Autodesk Fusion 360 part; units mm, degrees
(part 2 of 2)
  line L116 (-3.5026, 1.8837) -> (-3.7861, 1.7498)
  spline S162 degree 3 poles (-3.7861, 1.7498) (-3.7959, 1.7453) (-3.8154, 1.7365) (-3.8466, 1.7281) (-3.8788, 1.7224) (-3.9007, 1.7217) (-3.9118, 1.7214) knots 0 0 0 0 0.247984 0.494414 0.743586 1 1 1 1
  spline S163 degree 3 poles (-3.9118, 1.7214) (-3.9227, 1.7218) (-3.9444, 1.7224) (-3.9762, 1.728) (-4.0074, 1.7366) (-4.0269, 1.7453) (-4.0368, 1.7498) knots 0 0 0 0 0.252584 0.503062 0.749123 1 1 1 1
  line L117 (-4.0368, 1.7498) -> (-4.3174, 1.8837)
  spline S164 degree 3 poles (-4.3174, 1.8837) (-4.3247, 1.8874) (-4.3389, 1.8946) (-4.3581, 1.908) (-4.3741, 1.9236) (-4.3872, 1.941) (-4.3978, 1.9602) (-4.4047, 1.9815) (-4.4094, 2.0044) (-4.4098, 2.0204) (-4.41, 2.0286) knots 0 0 0 0 0.13429 0.261241 0.382043 0.499668 0.617596 0.738755 0.865582 1 1 1 1
  spline S165 degree 3 poles (-4.41, 2.0286) (-4.4097, 2.0365) (-4.4092, 2.052) (-4.4041, 2.0747) (-4.3958, 2.0962) (-4.3841, 2.1161) (-4.3702, 2.1342) (-4.3543, 2.1501) (-4.3369, 2.1637) (-4.3239, 2.1706) (-4.3174, 2.1741) knots 0 0 0 0 0.130456 0.256197 0.381397 0.509042 0.63603 0.7576 0.878449 1 1 1 1
  line L118 (-4.3174, 2.1741) -> (-4.0368, 2.3089)
  spline S166 degree 3 poles (-4.0368, 2.3089) (-4.0274, 2.313) (-4.0084, 2.3213) (-3.9779, 2.3297) (-3.9454, 2.3346) (-3.9232, 2.3354) (-3.9118, 2.3357) knots 0 0 0 0 0.237707 0.4823 0.734621 1 1 1 1
  spline S167 degree 3 poles (-3.9118, 2.3357) (-3.9004, 2.3354) (-3.8781, 2.3346) (-3.8456, 2.3297) (-3.8149, 2.3213) (-3.7956, 2.313) (-3.7861, 2.3089) knots 0 0 0 0 0.26409 0.515187 0.760253 1 1 1 1
  line L119 (-3.7861, 2.3089) -> (-3.5026, 2.1741)
  spline S168 degree 3 poles (6.6853, 3.6915) (6.6896, 3.6913) (6.6982, 3.691) (6.7104, 3.6872) (6.7215, 3.6813) (6.7315, 3.6733) (6.7397, 3.6636) (6.7457, 3.6526) (6.7494, 3.6406) (6.7498, 3.6322) (6.75, 3.6279) knots 0 0 0 0 0.128711 0.253233 0.375876 0.503288 0.630394 0.751088 0.873492 1 1 1 1
  spline S169 degree 3 poles (6.75, 3.6279) (6.7498, 3.6236) (6.7494, 3.6152) (6.7457, 3.6032) (6.7397, 3.5922) (6.7315, 3.5825) (6.7215, 3.5745) (6.7104, 3.5686) (6.6982, 3.5648) (6.6896, 3.5645) (6.6853, 3.5643) knots 0 0 0 0 0.126508 0.248912 0.369606 0.496712 0.624124 0.746767 0.871289 1 1 1 1
  line L120 (6.6853, 3.5643) -> (6.4527, 3.5643)
  line L121 (6.4527, 3.5643) -> (5.7962, 3.8156)
  spline S170 degree 3 poles (5.7962, 3.8156) (5.7925, 3.8173) (5.7855, 3.8206) (5.7759, 3.8266) (5.768, 3.8337) (5.7615, 3.8413) (5.7562, 3.8496) (5.7527, 3.8587) (5.7503, 3.8685) (5.7501, 3.8753) (5.75, 3.8788) knots 0 0 0 0 0.145956 0.279521 0.404592 0.524134 0.640675 0.75592 0.874017 1 1 1 1
  spline S171 degree 3 poles (5.75, 3.8788) (5.7501, 3.8825) (5.7503, 3.8896) (5.7527, 3.8998) (5.7562, 3.9093) (5.7614, 3.9178) (5.768, 3.9255) (5.7759, 3.9325) (5.7854, 3.9386) (5.7925, 3.9417) (5.7962, 3.9433) knots 0 0 0 0 0.12917 0.250463 0.368721 0.485595 0.603177 0.726199 0.857574 1 1 1 1
  line L122 (5.7962, 3.9433) -> (6.4527, 4.1929)
  line L123 (6.4527, 4.1929) -> (6.6853, 4.1929)
  spline S172 degree 3 poles (6.6853, 4.1929) (6.6896, 4.1927) (6.6982, 4.1923) (6.7104, 4.1886) (6.7216, 4.1826) (6.7315, 4.1746) (6.7398, 4.1649) (6.7456, 4.1537) (6.7495, 4.1416) (6.7498, 4.1331) (6.75, 4.1288) knots 0 0 0 0 0.128179 0.252186 0.374322 0.501208 0.627788 0.749924 0.871821 1 1 1 1
  spline S173 degree 3 poles (6.75, 4.1288) (6.7498, 4.1245) (6.7495, 4.116) (6.7457, 4.1039) (6.7398, 4.0929) (6.7315, 4.0832) (6.7216, 4.075) (6.7104, 4.069) (6.6982, 4.0653) (6.6896, 4.0649) (6.6853, 4.0647) knots 0 0 0 0 0.12825 0.250215 0.370477 0.497127 0.625471 0.747675 0.87175 1 1 1 1
  line L124 (6.6853, 4.0647) -> (6.4788, 4.0647)
  line L125 (6.4788, 4.0647) -> (5.9888, 3.8786)
  line L126 (5.9888, 3.8786) -> (6.4772, 3.6915)
  line L127 (6.4772, 3.6915) -> (6.6853, 3.6915)
  circle A8 centre (-5.7, -4.35) radius 1.5
  circle A9 centre (5.7, -4.35) radius 1.5
  line L128 (8.2, 7.85) -> (-8.2, 7.85)
  line L129 (-9.2, 6.85) -> (-9.2, -5.35)
  line L130 (-2.5, -13.15) -> (2.5, -13.15)
  line L131 (-8.2, 7.85) -> (-9.2, 7.85)
  line L132 (-9.2, 7.85) -> (-9.2, 6.85)
  line L133 (-9.2, 7.85) -> (9.3388, 7.85)
  line L134 (9.3388, 7.85) -> (9.3388, -13.0599)
  line L135 (9.3388, -13.0599) -> (-9.2, -13.0599)
  line L136 (-9.2, -13.0599) -> (-9.2, 7.85)
  line L137 (0, -11.7) -> (1.5, -11.7)
  line L138 (1.5, -11.7) -> (1.5, -8.6)
  line L139 (1.5, -8.6) -> (-1.5, -8.6)
  line L140 (-1.5, -8.6) -> (-1.5, -11.7)
  line L141 (-1.5, -11.7) -> (0, -11.7)
  dimension "d1" = 1
  dimension "d2" = 1
  dimension "d3" = 1
  constraint parallel L128 L131
  constraint horizontal L133
  constraint vertical L134
  constraint horizontal L135
  constraint vertical L136
  constraint perpendicular L9 L138
  constraint perpendicular L138 L139
  constraint perpendicular L9 L140
extrude "Extrusão1" add sketch "Esboço1" along normal blind 1 contours L0 A0 L1 L2 L3 L4 L5 L6 L7 A1 L8 L9 | A2 | A3 | A4 | A5 | A6 | A7 | S0 S1 L10 S2 L11 S3 S4 L12 S5 L13 S6 S7 L14 L15 L16 | S8 S9 L17 S10 S11 S12 L18 S13 S14 L19 S15 S16 L20 S17 S18 S19 S20 L21 S21 S22 L22 | L23 S23 L24 S24 S25 L25 S26 L26 S27 S28 L27 S29 L28 S30 S31 L29 S32 L30 S33 S34 | S35 L31 L32 S36 S37 L33 L34 S38 | S39 S40 L35 L36 L37 L38 S41 S42 L39 L40 L41 L42 | L43 S43 L44 S44 S45 L45 S46 L46 S47 L47 S48 L48 S49 L49 L50 S50 S51 L51 L52 S52 L53 S53 L54 S54 | L55 S55 L56 S56 S57 L57 S58 L58 S59 S60 L59 S61 L60 S62 S63 L61 S64 L62 S65 S66 | L63 S67 L64 S68 S69 L65 S70 L66 S71 S72 L67 S73 L68 S74 S75 L69 S76 L70 S77 S78 | S79 S80 L71 S81 S82 S83 L72 S84 S85 L73 S86 S87 L74 S88 S89 S90 S91 L75 S92 S93 L76 | L77 S94 L78 S95 S96 L79 S97 L80 S98 S99 L81 S100 L82 S101 S102 L83 S103 L84 S104 S105 | S106 S107 L85 S108 L86 S109 S110 L87 S111 L88 S112 S113 L89 L90 L91 | S114 S115 L92 S116 S117 S118 L93 S119 S120 L94 S121 S122 L95 S123 S124 S125 S126 L96 S127 S128 L97 | S129 S130 L98 S131 S132 L99 S133 S134 S135 L100 L101 L102 S136 | S137 S138 L103 S139 S140 S141 L104 S142 S143 L105 S144 S145 L106 S146 S147 S148 S149 L107 S150 S151 L108 | S152 S153 L109 S154 L110 S155 S156 L111 S157 L112 S158 S159 L113 L114 L115 | S160 S161 L116 S162 S163 L117 S164 S165 L118 S166 S167 L119 | S168 S169 L120 L121 S170 S171 L122 L123 S172 S173 L124 L125 L126 L127 | A8 | A9 | L128 L129 L131 L132 L133 L134 L135 L136 makes body 1
move_body "Mover1" bodies 1 to x (1, 0, 0) y (0, 1, 0) z (0, 0, 1) at (0, 1, 0)
sketch "Esboço2" plane through (0, 1.8, 0) normal (0, -1, 0) x (1, 0, 0)
  line L0 (1.5, -11.7) -> (-1.5, -11.7)
  line L1 (-1.5, -11.7) -> (-1.5, -8.6)
  line L2 (-1.5, -8.6) -> (1.5, -8.6)
  line L3 (1.5, -8.6) -> (1.5, -11.7)
  line L4 (-9.3388, -13.0599) -> (9.2, -13.0599)
  line L5 (9.2, -13.0599) -> (9.2, 7.85)
  line L6 (9.2, 7.85) -> (-9.3388, 7.85)
  line L7 (-9.3388, 7.85) -> (-9.3388, -13.0599)
  line L8 (10.2, 8.85) -> (-10.3388, 8.85)
  line L9 (-10.3388, 8.85) -> (-10.3388, -14.0599)
  line L10 (-10.3388, -14.0599) -> (10.2, -14.0599)
  line L11 (10.2, -14.0599) -> (10.2, 8.85)
  dimension "d6" = 1
extrude "Extrusão2" add sketch "Esboço2" against normal blind 1 contours L8 L9 L10 L11 bodies 1
sketch "Esboço3" plane through (0, 1.8, 0) normal (0, -1, 0) x (1, 0, 0)
  line L0 (10.2, -14.0599) -> (10.2, 8.85)
  line L1 (10.2, 8.85) -> (-10.3388, 8.85)
  line L2 (-10.3388, 8.85) -> (-10.3388, -14.0599)
  line L3 (-10.3388, -14.0599) -> (10.2, -14.0599)
  line L4 (1.5, -11.7) -> (-1.5, -11.7)
  line L5 (-1.5, -11.7) -> (-1.5, -8.6)
  line L6 (-1.5, -8.6) -> (1.5, -8.6)
  line L7 (1.5, -8.6) -> (1.5, -11.7)
  line L8 (9.2, 7.85) -> (-9.3388, 7.85)
  line L9 (-9.3388, 7.85) -> (-9.3388, -13.0599)
  line L10 (-9.3388, -13.0599) -> (9.2, -13.0599)
  line L11 (9.2, -13.0599) -> (9.2, 7.85)
  dimension "d9" = -1
extrude "Extrusão3" add sketch "Esboço3" along normal blind 4 contours L0 L1 L2 L3 bodies 1
sketch "Esboço4" plane through (0, -2.2, 0) normal (0, -1, 0) x (1, 0, 0)
  line L0 (9.2, 7.85) -> (9.2, -13.0599)
  line L1 (9.2, -13.0599) -> (-9.3388, -13.0599)
  line L2 (-9.3388, -13.0599) -> (-9.3388, 7.85)
  line L3 (-9.3388, 7.85) -> (9.2, 7.85)
  line L4 (-10.3388, -14.0599) -> (10.2, -14.0599)
  line L5 (10.2, -14.0599) -> (10.2, 8.85)
  line L6 (10.2, 8.85) -> (-10.3388, 8.85)
  line L7 (-10.3388, 8.85) -> (-10.3388, -14.0599)
  line L8 (9.2, 4.2997) -> (-9.3388, 4.2997)
  line L9 (-9.3388, 4.2997) -> (-9.3388, -13.0599)
  line L10 (-9.3388, -13.0599) -> (9.2, -13.0599)
  line L11 (9.2, 4.2997) -> (9.2, -13.0599)
  constraint coincident L0 L8.start
  constraint coincident L2 L8.end
  constraint perpendicular L2 L8
  constraint coincident L1.end L2.start
  constraint perpendicular L1 L9
  constraint coincident L0.end L1.start
extrude "Extrusão4" add sketch "Esboço4" against normal blind 1 contours L0 L1 L2 L8 L9 L10 L11 bodies 1
sketch "Esboço5" plane through (0, 2.8, 0) normal (0, 1, 0) x (-1, 0, 0)
  line L0 (-10.2, 8.85) -> (-10.2, -14.0599)
  line L1 (-10.2, -14.0599) -> (10.3388, -14.0599)
  line L2 (10.3388, -14.0599) -> (10.3388, 8.85)
  line L3 (10.3388, 8.85) -> (-10.2, 8.85)
  line L4 (1.5, -11.7) -> (-1.5, -11.7)
  line L5 (-1.5, -11.7) -> (-1.5, -8.6)
  line L6 (-1.5, -8.6) -> (1.5, -8.6)
  line L7 (1.5, -8.6) -> (1.5, -11.7)
  line L8 (9.3388, 7.85) -> (-9.2, 7.85)
  line L9 (-9.2, 7.85) -> (-9.2, -13.0599)
  line L10 (-9.2, -13.0599) -> (9.3388, -13.0599)
  line L11 (9.3388, -13.0599) -> (9.3388, 7.85)
  dimension "d14" = -1
extrude "Extrusão1'" add sketch "Esboço5" along normal blind 1 separate body contours L8 L9 L10 L11 makes body 2 in component "Component"
sketch "Esboço6" plane through (0, 2.8, 0) normal (0, 1, 0) x (-1, 0, 0)
  line L0 (-10.2, 8.85) -> (-10.2, -14.0599)
  line L1 (-10.2, -14.0599) -> (10.3388, -14.0599)
  line L2 (10.3388, -14.0599) -> (10.3388, 8.85)
  line L3 (10.3388, 8.85) -> (-10.2, 8.85)
  line L4 (1.5, -11.7) -> (-1.5, -11.7)
  line L5 (-1.5, -11.7) -> (-1.5, -8.6)
  line L6 (-1.5, -8.6) -> (1.5, -8.6)
  line L7 (1.5, -8.6) -> (1.5, -11.7)
  line L8 (9.3388, 7.85) -> (-9.2, 7.85)
  line L9 (-9.2, 7.85) -> (-9.2, -13.0599)
  line L10 (-9.2, -13.0599) -> (9.3388, -13.0599)
  line L11 (9.3388, -13.0599) -> (9.3388, 7.85)
  dimension "d17" = -1
extrude "Extrusão5" cut sketch "Esboço6" against normal blind 1 contours L8 L9 L10 L11 bodies 1
sketch "Esboço7" plane through (0, 0, -13.0599) normal (0, 0, 1) x (-1, 0, 0)
  line L0 (9.3388, 1.2) -> (-9.2, 1.2)
  line L1 (-9.2, 1.2) -> (-9.2, -2.8)
  line L2 (-9.2, -2.8) -> (9.3388, -2.8)
  line L3 (9.3388, -2.8) -> (9.3388, 1.2)
  line L4 (9.3388, -2.8) -> (9.3388, -1.8)
  line L5 (9.3388, -1.8) -> (9.3388, -0.8)
  line L6 (9.3388, -1.8) -> (-9.2, -1.8)
  line L7 (9.3388, -0.8) -> (-9.2, -0.8)
  line L8 (-9.2, -1.8) -> (-9.2, -0.8)
  dimension "d20" = 1
  constraint coincident L2.end L3.start
  constraint perpendicular L2 L4
  constraint midpoint L3 L5.end
  constraint coincident L1 L6.end
  constraint perpendicular L1 L6
  constraint midpoint L1 L7.end
  measures "d20" distance of L2.end L4.end
extrude "Extrusão6" add sketch "Esboço7" along normal blind 21.9099 contours L1 L3 L5 L6 L7 L8 bodies 1
sketch "Esboço8" plane through (0, 1.8, 0) normal (0, 1, 0) x (-1, 0, 0)
  line L0 (9.3388, 7.85) -> (-9.2, 7.85)
  line L1 (-9.2, 7.85) -> (-9.2, -13.0599)
  line L2 (-9.2, -13.0599) -> (9.3388, -13.0599)
  line L3 (9.3388, -13.0599) -> (9.3388, 7.85)
  line L4 (8.3388, 6.85) -> (-8.2, 6.85)
  line L5 (-8.2, 6.85) -> (-8.2, -12.0599)
  line L6 (-8.2, -12.0599) -> (8.3388, -12.0599)
  line L7 (8.3388, -12.0599) -> (8.3388, 6.85)
  dimension "d23" = -1
extrude "Extrusão7" cut sketch "Esboço8" against normal blind 1 contours L4 L5 L6 L7 bodies 1
move_face "Deslocar faces1" offset 1 1 faces at (-3.1592, -2.2, -7.9401) on bodies 1
extrude "Extrusão8" cut 1 faces at (-3.1592, -1.2, -1.4869) along direction (0, -1, 0) blind 1 on bodies 1 bodies 1
component "Component" placed x (1, 0, 0) y (0, 1, 0) z (0, 0, 1) at (0, 32, 0)
